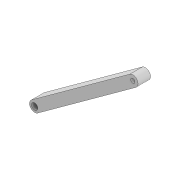
# Autodesk Inventor part: Second part of arm of gripper
Saved by Autodesk Inventor 2020.3 (Build 243373010, 373A)
## iProperties
Created: 2021-05-15
Part Number: Second part of arm of gripper
Material: Generic
Document SubType Name: Modeling
Designer: marti
Density: 1 g/cm^3
Appearance: Default
Author: marti
Autodesk Inventor part; units mm, degrees
ref_plane "YZ Plane" through (0, 0, 0) normal (1, 0, 0) x (0, 1, 0)
ref_plane "XZ Plane" through (0, 0, 0) normal (0, 1, 0) x (-1, 0, 0)
ref_plane "XY Plane" through (0, 0, 0) normal (0, 0, 1) x (1, 0, 0)
sketch "Sketch1" plane through (0, 0, 0) normal (0, 0, 1) x (1, 0, 0)
  arc A0 (-142.7162, -169.544) -> (-130.9605, -185.7243) centre (-136.8383, -177.6341) ccw
  line L0 (-17.6981, -103.4344) -> (-130.9605, -185.7243)
  line L1 (46.5951, -32.0012) -> (-142.7162, -169.544)
  line L2 (-17.6981, -103.4344) -> (58.3508, -48.1816)
  arc A1 (58.3508, -48.1816) -> (46.5951, -32.0012) centre (52.473, -40.0914) ccw
  circle A2 centre (52.473, -40.0914) radius 4
  circle A3 centre (-136.8383, -177.6341) radius 6
  point P0 (0, 0)
  point P1 (0, 0)
  dimension "d0" = 8
  dimension "d3" = 12
  constraints: 6 end point, 4 centre point, 4 point on circle, 2 coincident, 1 other
  measures "d0" diameter of A2
  measures "d3" diameter of A3
extrude "Extrusion1" add sketch "Sketch1" along normal mid plane 24
body "Solid1"
